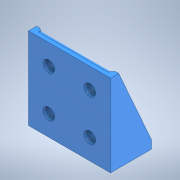
# Autodesk Inventor part: Bottom_Bracket
Saved by Autodesk Inventor 2021 (Build 250183000, 183)
## iProperties
Created: 2021-05-04
Part Number: Bottom_Bracket
Material: Generic
Document SubType Name: Modeling
Designer: Jorian Brusind
Density: 1 g/cm^3
Appearance: Cyan
Author: Jorian Brusind
Autodesk Inventor part; units mm, degrees
ref_plane "YZ Plane" through (0, 0, 0) normal (1, 0, 0) x (0, 1, 0)
ref_plane "XZ Plane" through (0, 0, 0) normal (0, 1, 0) x (-1, 0, 0)
ref_plane "XY Plane" through (0, 0, 0) normal (0, 0, 1) x (1, 0, 0)
sketch "Sketch1" plane through (0, 0, 0) normal (0, 1, 0) x (-1, 0, 0)
  line L0 (0, 0) -> (40, 0)
  line L1 (40, 0) -> (40, -20)
  line L2 (40, -20) -> (0, -20)
  line L3 (0, -20) -> (0, 0)
  dimension "d0" = 40
  dimension "d1" = 20
  constraints: 8 end point, 2 parallel, 1 horizontal, 1 perpendicular
  measures "d0" distance of L1.end L2.end
  measures "d1" distance of L0.end L1.end
extrude "Extrusion1" add sketch "Sketch1" along normal blind 4
sketch "Sketch2" plane through (0, 4, 0) normal (0, 1, 0) x (1, 0, 0)
  circle A0 centre (-30, 10) radius 2.75
  circle A1 centre (-10, 10) radius 2.75
  line L0 (0, 20) -> (-40, 20) projected
  line L1 (-40, 20) -> (-40, 0) projected
  point P0 (0, 0)
  dimension "d4" = 5.5
  dimension "d5" = 5.5
  dimension "d6" = 10
  dimension "d7" = 10
  dimension "d8" = 20
  constraints: 2 centre point, 1 horizontal alignment
  measures "d4" diameter of A0
  measures "d5" diameter of A1
  measures "d6" distance from line of L0 A0.centre
  measures "d7" distance from line of L1 A0.centre
  measures "d8" distance of A0.centre A1.centre
extrude "Extrusion2" cut sketch "Sketch2" against normal through all
sketch "Sketch3" plane through (0, 4, 0) normal (0, 1, 0) x (1, 0, 0)
  line L0 (-40, 20) -> (-40, 0) projected
  line L1 (-40, 0) -> (0, 0)
  line L2 (0, 0) -> (0, 4)
  line L3 (0, 4) -> (-40, 4)
  line L4 (-40, 4) -> (-40, 0)
  dimension "d11" = 40
  dimension "d12" = 4
  constraints: 8 end point, 2 parallel, 1 horizontal, 1 perpendicular
  measures "d11" distance of L3.end L2.end
  measures "d12" distance of L2.end L1.end
extrude "Extrusion3" add sketch "Sketch3" along normal blind 36
sketch "Sketch4" plane through (0, 4, -4) normal (0, 0, -1) x (-1, 0, 0)
  circle A0 centre (10, 26) radius 2.75
  line L0 (0, 0) -> (0, 36) projected
  line L1 (0, 36) -> (40, 36) projected
  point P0 (0, -4)
  dimension "d15" = 5.5
  dimension "d16" = 10
  dimension "d17" = 10
  constraints: 1 centre point
  measures "d15" diameter of A0
  measures "d16" distance from line of L0 A0.centre
  measures "d17" distance from line of L1 A0.centre
extrude "Extrusion4" cut sketch "Sketch4" against normal through all
pattern_linear "Rectangular Pattern1" count 2 spacing 20 along (0, -1, 0) count 2 spacing 20 along (-1, 0, 0) of "Extrusion4"
sketch "Sketch5" plane through (0, 0, 0) normal (1, 0, 0) x (0, 0, -1)
  line L0 (4, 4) -> (4, 40) projected
  line L1 (20, 4) -> (4, 4) projected
  line L2 (4, 40) -> (20, 4)
  line L3 (20, 4) -> (4, 4)
  line L4 (4, 4) -> (4, 40)
  point P0 (0, 0)
  constraints: 6 end point, 1 collinear, 1 perpendicular
extrude "Extrusion5" add sketch "Sketch5" against normal blind 3
pattern_linear "Rectangular Pattern2" count 2 spacing 37 along (-1, 0, 0) of "Extrusion5"
fillet "Fillet1" radius 2 4 edges at (-20, 4, -20) (-20, 40, -4) (-3, 22, -12) (-37, 22, -12)
body "Solid1"
